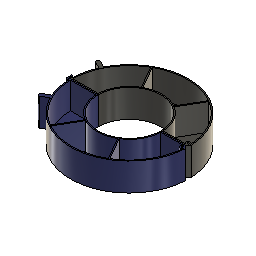
Day15 - Box with BCN3D spools continued (Autodesk Fusion 360 design; units mm, degrees)
Autodesk Fusion 360 part; units mm, degrees
note: some values were not read from the file. Set by a fixed rule: which sketch regions a step uses.
sketch "Sketch1" plane through (0, 0, 0) normal (0, 0, 1) x (1, 0, 0)
  arc A0 (100, 0) -> (-100, 0) centre (0, 0) ccw
  line L0 (0, 0) -> (100, 0) construction
  line L1 (0, 0) -> (-100, 0) construction
  arc A1 (53, 0) -> (-53, 0) centre (0, 0) ccw
  line L2 (0, 0) -> (53, 0) construction
  line L3 (0, 0) -> (-53, 0) construction
  line L4 (-100, 0) -> (-53, 0)
  line L5 (53, 0) -> (100, 0)
  line L6 (94.399, 0) -> (99.8513, 5.4523)
  line L7 (94.399, 0) -> (102.1097, 0) construction
  line L8 (-89.1925, 45.2184) -> (-102.7789, 52.5129)
  line L9 (-102.7789, 52.5129) -> (-105.6171, 47.2267)
  line L10 (-105.6171, 47.2267) -> (-91.7472, 39.78)
  circle A2 centre (94.5188, 5.0696) radius 1.5
  circle A3 centre (94.5188, 5.0696) radius 2.5
  line L11 (0, 0) -> (-50, 86.6025)
  line L12 (0, 0) -> (50, 86.6025)
  line L13 (1.7321, 1) -> (-48.2679, 87.6025)
  line L14 (1.7321, -1) -> (51.7321, 85.6025)
  dimension "d1" = 100
  dimension "d5" = 47
  dimension "d6" = 45
  dimension "d7" = 6
  dimension "d11" = 3
  dimension "d12" = 2
  dimension "d13" = 5
  dimension "d25" = 60
  dimension "d26" = 60
  dimension "d27" = 2
  dimension "d28" = 2
  measures "d1" radius of A0
  measures "d5" distance of A0 A1
  measures "d6" angle of L6 L7
  measures "d11" diameter of A2
  measures "d13" diameter of A3
  measures "d25" angle of L1 L11
  measures "d26" angle of L2 L12
extrude "Extrude1" add sketch "Sketch1" along normal blind 47 contours A0 A1 L5 L6 L14 | A0 A1 L12 L14 | A0 A1 L12 L13 | A0 A1 L11 L13 | A0 A1 L4 L11 | A3 makes body 1
shell "Shell1" thickness 2 removed faces 1 at (80.8693, 23.265, 47) on bodies 1
extrude "Extrude2" add sketch "Sketch1" along normal up to surface (47 mm away) contours A0 L8 L9 L10 bodies 1
extrude "Extrude5" add sketch "Sketch1" along normal up to surface (47 mm away) contours A0 A1 L12 L14 | A0 A1 L11 L13 bodies 1
mirror "Mirror1" about plane through (0, 0, 0) normal (0, 1, 0) of bodies 1 makes body 2
sketch "Sketch2" plane through (0, 0, 0) normal (0, 0, 1) x (1, 0, 0)
  arc A0 (100, 0) -> (-100, 0) centre (0, 0) ccw
  arc A1 (-100, 0) -> (-91.7472, -39.78) centre (0, 0) ccw
  arc A2 (-99.3608, 3.8951) -> (-100, 0) centre (-100, 2) ccw
  line L0 (-100, 0) -> (-102.7643, 0)
  line L1 (-102.7643, 0) -> (-102.7643, 2.9485)
  arc A3 (-99.8526, 5.4275) -> (-99.8385, 5.6804) centre (-101.6525, 5.6545) ccw
  arc A4 (-102.7643, 2.9485) -> (-103.3053, 6.8739) centre (-103.3053, 4.8739) ccw
  line L2 (-103.3053, 6.8739) -> (-104.7643, 6.8739)
  line L3 (-104.7643, 6.8739) -> (-104.7643, -3.198)
  line L4 (-104.7643, -3.198) -> (-99.9489, -3.198)
  line L5 (-100, 0) -> (-53, 0)
  dimension "d17" = 2
  dimension "d18" = 2
  dimension "d19" = 2
  measures "d17" distance of L1 L3
  measures "d18" radius of A2
  measures "d19" radius of A4
extrude "Extrude3" add sketch "Sketch2" along normal up to surface (47 mm away) separate body contours A1 L0 L1 A4 L2 L3 L4 makes body 3
extrude "Extrude4" add sketch "Sketch2" along normal up to surface (47 mm away) separate body contours A0 A2 makes body 4
combine "Combine1" operation add target body 4 tool bodies 1
combine "Combine2" operation add target body 2 tool bodies 3
fillet "Fillet1" radius 2 5 edges at (-102.7789, -52.5129, 23.5) (-105.6171, -47.2267, 23.5) (-104.7643, -3.198, 23.5) (-105.6171, 47.2267, 23.5) (-102.7789, 52.5129, 23.5) on bodies 2 4
